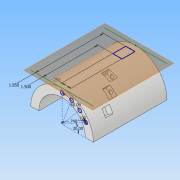
# Autodesk Inventor part: Core
Saved by Autodesk Inventor 2017.3 (Build 213256000, 256)
## iProperties
Created: 2019-05-16
Part Number: Core
Material: ABS Plastic
Document SubType Name: Modeling
Designer: Derek Wider
Density: 1.06 g/cm^3
Appearance: Smooth - White
Author: Derek Wider
Autodesk Inventor part; units mm, degrees
ref_plane "YZ Plane" through (0, 0, 0) normal (1, 0, 0) x (0, 1, 0)
ref_plane "XZ Plane" through (0, 0, 0) normal (0, 1, 0) x (-1, 0, 0)
ref_plane "XY Plane" through (0, 0, 0) normal (0, 0, 1) x (1, 0, 0)
sketch "Sketch1" plane through (0, 0, 0) normal (0, 0, 1) x (1, 0, 0)
  arc A0 (16.002, 0) -> (-16.002, 0) centre (0, 0) ccw
  arc A1 (21.59, 0) -> (-21.59, 0) centre (0, 0) ccw
  line L0 (-16.002, 0) -> (-21.59, 0)
  line L1 (16.002, 0) -> (21.59, 0)
  dimension "d0" = 32.004
  dimension "d1" = 43.18
  constraints: 4 end point, 4 point on circle, 2 centre point, 2 coincident, 2 point on line, 1 horizontal
  measures "d0" diameter of A0
  measures "d1" diameter of A1
extrude "Extrusion1" add sketch "Sketch1" along normal blind 50.8
sketch "Sketch2" plane through (0, 0, 50.8) normal (0, 0, 1) x (1, 0, 0)
  circle A0 centre (16.2778, 9.398) radius 1.27
  line L0 (0, 0) -> (16.2778, 9.398) construction
  line L1 (0, 0) -> (18.796, 0) construction
  circle A1 centre (12.0818, 14.3986) radius 1.27
  circle A2 centre (6.4286, 17.6625) radius 1.27
  circle A3 centre (0, 18.796) radius 1.27
  line L2 (0, 0) -> (12.0818, 14.3986) construction
  line L3 (0, 0) -> (6.4286, 17.6625) construction
  line L4 (0, 0) -> (0, 18.796) construction
  dimension "d4" = 2.54
  dimension "d5" = 18.796
  dimension "d6" = 30
  dimension "d9" = 60
  constraints: 10 end point, 4 centre point, 1 coincident, 1 equal length, 1 horizontal, 7 other
  measures "d4" diameter of A0
  measures "d5" distance of L0.start L0.end
  measures "d6" angle of L1 L0
extrude "Extrusion2" cut sketch "Sketch2" against normal blind 12.7 contours A0
extrude "Extrusion3" cut sketch "Sketch2" against normal blind 25.4 contours A1
extrude "Extrusion4" cut sketch "Sketch2" against normal blind 31.75 contours A2
extrude "Extrusion5" cut sketch "Sketch2" against normal blind 38.1 contours A3
ref_plane "Work Plane4" through (18.6975, 10.795, 0) normal (0.8660254, 0.5, 0) x (-0.5, 0.8660254, 0)
ref_plane "Work Plane3" through (16.2778, 9.398, 50.8) normal (0.8660254, 0.5, 0) x (-0.5, 0.8660254, 0)
sketch "Sketch3" plane through (18.6975, 10.795, 0) normal (0.8660254, 0.5, 0) x (-0.5, 0.8660254, 0)
  line L0 (2.54, 40.64) -> (-2.54, 40.64)
  line L1 (-2.54, 40.64) -> (-2.54, 35.56)
  line L2 (-2.54, 35.56) -> (2.54, 35.56)
  line L3 (2.54, 35.56) -> (2.54, 40.64)
  line L4 (21.59, 50.8) -> (-10.795, 50.8) projected
  point P0 (0, 0)
  point P1 (10.795, 50.8)
  point P2 (0, 35.56)
  dimension "d20" = 10.16
  dimension "d21" = 15.24
  dimension "d22" = 5.08
  constraints: 8 end point, 2 parallel, 1 horizontal, 1 midpoint, 1 perpendicular, 1 vertical alignment
  measures "d20" distance between parallel lines of L4 L0
  measures "d21" distance between parallel lines of L4 L2
  measures "d22" distance between parallel lines of L3 L1
extrude "Extrusion6" cut sketch "Sketch3" against normal blind 4.318
ref_plane "Work Plane7" through (13.8778, 16.5389, 0) normal (0.6427876, 0.7660444, 0) x (-0.7660444, 0.6427876, 0)
ref_plane "Work Plane6" through (12.0818, 14.3986, 50.8) normal (0.6427876, 0.7660444, 0) x (-0.7660444, 0.6427876, 0)
sketch "Sketch4" plane through (13.8778, 16.5389, 0) normal (0.6427876, 0.7660444, 0) x (-0.7660444, 0.6427876, 0)
  line L0 (3.175, 34.29) -> (-3.175, 34.29)
  line L1 (-3.175, 34.29) -> (-3.175, 29.21)
  line L2 (-3.175, 29.21) -> (3.175, 29.21)
  line L3 (3.175, 29.21) -> (3.175, 34.29)
  line L4 (21.59, 50.8) -> (-16.5389, 50.8) projected
  point P0 (0, 0)
  point P1 (0, 29.21)
  point P2 (16.5389, 50.8)
  dimension "d25" = 6.35
  dimension "d26" = 16.51
  dimension "d27" = 21.59
  constraints: 8 end point, 2 parallel, 1 horizontal, 1 midpoint, 1 perpendicular, 1 vertical alignment
  measures "d25" distance of L0.start L0.end
  measures "d26" distance between parallel lines of L4 L0
  measures "d27" distance between parallel lines of L4 L2
extrude "Extrusion7" cut sketch "Sketch4" against normal blind 4.318
ref_plane "Work Plane9" through (7.3842, 20.288, 0) normal (0.3420201, 0.9396926, 0) x (-0.9396926, 0.3420201, 0)
ref_plane "Work Plane8" through (6.4286, 17.6625, 50.8) normal (0.3420201, 0.9396926, 0) x (-0.9396926, 0.3420201, 0)
sketch "Sketch5" plane through (7.3842, 20.288, 0) normal (0.3420201, 0.9396926, 0) x (-0.9396926, 0.3420201, 0)
  line L0 (-3.175, 22.86) -> (3.175, 22.86)
  line L1 (3.175, 22.86) -> (3.175, 27.94)
  line L2 (3.175, 27.94) -> (-3.175, 27.94)
  line L3 (-3.175, 27.94) -> (-3.175, 22.86)
  line L4 (21.59, 50.8) -> (-20.288, 50.8) projected
  point P0 (0, 0)
  point P1 (20.288, 50.8)
  point P2 (0, 22.86)
  dimension "d30" = 6.35
  dimension "d31" = 22.86
  dimension "d32" = 27.94
  constraints: 8 end point, 2 parallel, 1 horizontal, 1 midpoint, 1 perpendicular, 1 vertical alignment
  measures "d30" distance of L1.end L2.end
  measures "d31" distance between parallel lines of L4 L2
  measures "d32" distance between parallel lines of L4 L0
extrude "Extrusion8" cut sketch "Sketch5" against normal blind 4.318
ref_plane "Work Plane11" through (0, 21.59, 0) normal (0, 1, 0) x (-1, 0, 0)
ref_plane "Work Plane10" through (0, 18.796, 50.8) normal (0, 1, 0) x (-1, 0, 0)
sketch "Sketch6" plane through (0, 21.59, 0) normal (0, 1, 0) x (-1, 0, 0)
  line L0 (3.175, 12.7) -> (-3.175, 12.7)
  line L1 (-3.175, 12.7) -> (-3.175, 3.81)
  line L2 (-3.175, 3.81) -> (3.175, 3.81)
  line L3 (3.175, 3.81) -> (3.175, 12.7)
  line L4 (21.59, 0) -> (-21.59, 0) projected
  line L5 (21.59, 50.8) -> (-21.59, 50.8) projected
  point P0 (0, 0)
  point P1 (0, 3.81)
  point P2 (0, 0)
  dimension "d35" = 6.35
  dimension "d36" = 38.1
  dimension "d37" = 46.99
  constraints: 8 end point, 2 midpoint, 2 parallel, 1 horizontal, 1 perpendicular, 1 vertical alignment
  measures "d35" distance of L0.start L0.end
  measures "d36" distance between parallel lines of L5 L0
  measures "d37" distance between parallel lines of L5 L2
body "Solid1"
